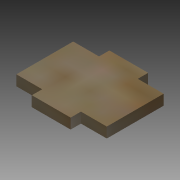
# Autodesk Inventor part: stubbur
Saved by Autodesk Inventor 2016 (Build 200138000, 138)
## iProperties
Created: 2015-10-06
Part Number: stubbur
Material: Generic
Document SubType Name: Modeling
Designer: Haukur
Density: 1 g/cm^3
Appearance: Plywood - Weathered
Author: Haukur
Autodesk Inventor part; units mm, degrees
ref_plane "YZ Plane" through (0, 0, 0) normal (1, 0, 0) x (0, 1, 0)
ref_plane "XZ Plane" through (0, 0, 0) normal (0, 1, 0) x (-1, 0, 0)
ref_plane "XY Plane" through (0, 0, 0) normal (0, 0, 1) x (1, 0, 0)
sketch "Sketch1" plane through (0, 0, 0) normal (0, 0, 1) x (1, 0, 0)
  line L0 (0, 4) -> (0, 26)
  line L1 (0, 26) -> (10, 26)
  line L2 (10, 26) -> (10, 30)
  line L3 (10, 30) -> (25, 30)
  line L4 (25, 30) -> (25, 26)
  line L5 (25, 26) -> (35, 26)
  line L6 (35, 26) -> (35, 4)
  line L7 (35, 4) -> (25, 4)
  line L8 (25, 4) -> (25, 0)
  line L9 (25, 0) -> (10, 0)
  line L10 (10, 0) -> (10, 4)
  line L11 (0, 4) -> (10, 4)
  point P0 (0, 0)
  dimension "d0" = 22
  dimension "d1" = 10
  dimension "d2" = 4
  dimension "d3" = 15
  dimension "d4" = 10
  dimension "d5" = 22
  constraints: 24 end point, 7 perpendicular, 7 point on line, 1 vertical
  measures "d0" distance of L0.start L0.end
  measures "d1" distance of L0.end L1.end
  measures "d2" distance of L1.end L2.end
  measures "d3" distance of L2.end L3.end
  measures "d4" distance of L4.end L5.end
  measures "d5" distance of L5.end L6.end
extrude "Extrusion1" add sketch "Sketch1" along normal blind 4
body "Solid1"
